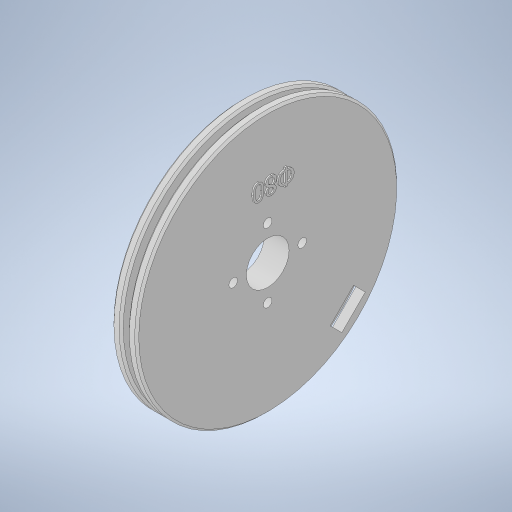
# Autodesk Inventor part: pully_shoulder_2_70
Saved by Autodesk Inventor 2024 (Build 280153000, 153)
## iProperties
Created: 2025-06-10
Part Number: pully_shoulder_2_70
Material: 一般
Document SubType Name: Modeling
Designer: HosodaLab2
Density: 1 g/cm^3
Appearance: 既定
Author: HosodaLab2
Autodesk Inventor part; units mm, degrees
ref_plane "YZ Plane" through (0, 0, 0) normal (1, 0, 0) x (0, 1, 0)
ref_plane "XZ Plane" through (0, 0, 0) normal (0, 1, 0) x (-1, 0, 0)
ref_plane "XY Plane" through (0, 0, 0) normal (0, 0, 1) x (1, 0, 0)
sketch "スケッチ1" plane through (0, 0, 0) normal (0, 1, 0) x (-1, 0, 0)
  circle A0 centre (0, 0) radius 40
  dimension "d0" = 80
  constraints: 1 centre point, 1 coincident
  measures "d0" diameter of A0
extrude "押し出し1" add sketch "スケッチ1" along normal blind 2.2
sketch "スケッチ2" plane through (0, 2.2, 0) normal (0, 1, 0) x (1, 0, 0)
  circle A0 centre (0, 0) radius 47.5
  line L0 (-3.6848, -24.5947) -> (4.9338, -24.5947) construction
  line L1 (4.9338, -24.5947) -> (4.9338, -28.142) construction
  line L2 (4.9338, -28.142) -> (-3.6848, -28.142) construction
  line L3 (-3.6848, -28.142) -> (-3.6848, -24.5947) construction
  dimension "d3" = 95
  constraints: 1 centre point, 1 coincident, 2 other
  measures "d3" diameter of A0
extrude "押し出し2" add sketch "スケッチ2" along normal blind 3.4
chamfer "面取り1" distance 0.75 angle 45 1 edges at (-47.5, 2.2, 0)
chamfer "面取り2" distance 0.75 angle 45 1 edges at (-47.5, 5.6, 0)
sketch "スケッチ3" plane through (0, 0, 0) normal (0, -1, 0) x (1, 0, 0)
  circle A0 centre (0, 0) radius 47.5
  dimension "d12" = 95
  constraints: 1 centre point, 1 coincident
  measures "d12" diameter of A0
extrude "押し出し3" add sketch "スケッチ3" along normal blind 3.4
chamfer "面取り3" distance 0.75 angle 45 1 edges at (-47.5, 0, 0)
chamfer "面取り4" distance 0.75 angle 45 1 edges at (-47.5, -3.4, 0)
sketch "スケッチ6" plane through (0, 5.6, 0) normal (0, 1, 0) x (1, 0, 0)
  circle A0 centre (0, 0) radius 7.65
  line L0 (0, 7.65) -> (46.8799, 7.65)
  circle A1 centre (0, 0) radius 47.5 projected
  line L1 (0, -7.65) -> (46.8799, -7.65)
  dimension "d39" = 15.3
  constraints: 4 end point, 4 point on circle, 1 centre point, 1 coincident, 1 horizontal, 1 parallel, 1 tangent
  measures "d39" diameter of A0
extrude "押し出し5" [suppressed]
chamfer "面取り7" [suppressed]
chamfer "面取り8" [suppressed]
chamfer "面取り9" [suppressed]
sketch "スケッチ7" plane through (0, 5.6, 0) normal (0, 1, 0) x (1, 0, 0)
  line L0 (-9.3358, -20.9354) -> (21.308, -20.9354) construction
  line L1 (21.308, -20.9354) -> (21.308, -27.5341) construction
  line L2 (21.308, -27.5341) -> (-9.3358, -27.5341) construction
  line L3 (-9.3358, -27.5341) -> (-9.3358, -20.9354) construction
  spline S0 degree 2 poles (-5.7914, -21.672) (-5.2131, -21.6818) (-4.2541, -22.0674) (-3.9377, -22.3887) knots 0 0 0 1 2 2 2
  spline S1 degree 2 poles (-3.9377, -22.3887) (-3.646, -22.6903) (-3.3247, -23.5356) (-3.3247, -24.0793) knots 0 0 0 1 2 2 2
  spline S2 degree 2 poles (-3.3247, -24.0793) (-3.3247, -24.6478) (-3.6708, -25.5228) (-3.9772, -25.8194) knots 0 0 0 1 2 2 2
  spline S3 degree 2 poles (-3.9772, -25.8194) (-4.3084, -26.1456) (-5.2773, -26.5065) (-5.7914, -26.5164) knots 0 0 0 1 2 2 2
  line L4 (-5.7914, -26.5164) -> (-5.7914, -27.2232)
  line L5 (-5.7914, -27.2232) -> (-6.6021, -27.2232)
  line L6 (-6.6021, -27.2232) -> (-6.6021, -26.5164)
  spline S4 degree 2 poles (-6.6021, -26.5164) (-7.1162, -26.5015) (-8.0802, -26.1654) (-8.4213, -25.8292) knots 0 0 0 1 2 2 2
  spline S5 degree 2 poles (-8.4213, -25.8292) (-8.7277, -25.5277) (-9.0688, -24.6429) (-9.0688, -24.0793) knots 0 0 0 1 2 2 2
  spline S6 degree 2 poles (-9.0688, -24.0793) (-9.0688, -23.5455) (-8.7426, -22.7002) (-8.446, -22.3937) knots 0 0 0 1 2 2 2
  spline S7 degree 2 poles (-8.446, -22.3937) (-8.1296, -22.0674) (-7.1805, -21.6868) (-6.6021, -21.672) knots 0 0 0 1 2 2 2
  line L7 (-6.6021, -21.672) -> (-6.6021, -21.0244)
  line L8 (-6.6021, -21.0244) -> (-5.7914, -21.0244)
  line L9 (-5.7914, -21.0244) -> (-5.7914, -21.672)
  spline S8 degree 2 poles (-5.7914, -25.9034) (-5.4207, -25.8935) (-4.8473, -25.6711) (-4.6594, -25.4832) knots 0 0 0 1 2 2 2
  spline S9 degree 2 poles (-4.6594, -25.4832) (-4.4073, -25.2361) (-4.17, -24.5292) (-4.17, -24.0447) knots 0 0 0 1 2 2 2
  spline S10 degree 2 poles (-4.17, -24.0447) (-4.17, -23.6394) (-4.3974, -22.972) (-4.6248, -22.7397) knots 0 0 0 1 2 2 2
  spline S11 degree 2 poles (-4.6248, -22.7397) (-4.8374, -22.5173) (-5.4009, -22.3047) (-5.7914, -22.2948) knots 0 0 0 1 2 2 2
  line L10 (-5.7914, -22.2948) -> (-5.7914, -25.9034)
  spline S12 degree 2 poles (-6.6021, -22.2948) (-6.9926, -22.2997) (-7.5562, -22.5222) (-7.7687, -22.7397) knots 0 0 0 1 2 2 2
  spline S13 degree 2 poles (-7.7687, -22.7397) (-7.9961, -22.9671) (-8.2235, -23.6493) (-8.2235, -24.0447) knots 0 0 0 1 2 2 2
  spline S14 degree 2 poles (-8.2235, -24.0447) (-8.2235, -24.5292) (-7.9862, -25.241) (-7.7341, -25.4832) knots 0 0 0 1 2 2 2
  spline S15 degree 2 poles (-7.7341, -25.4832) (-7.5463, -25.6612) (-6.9729, -25.8985) (-6.6021, -25.9034) knots 0 0 0 1 2 2 2
  line L11 (-6.6021, -25.9034) -> (-6.6021, -22.2948)
  spline S16 degree 2 poles (-0.7691, -27.3122) (-1.2238, -27.3122) (-1.9703, -27.0403) (-2.2323, -26.7882) knots 0 0 0 1 2 2 2
  spline S17 degree 2 poles (-2.2323, -26.7882) (-2.4893, -26.5411) (-2.7563, -25.8688) (-2.7563, -25.4882) knots 0 0 0 1 2 2 2
  spline S18 degree 2 poles (-2.7563, -25.4882) (-2.7563, -24.9938) (-2.2273, -24.1634) (-1.7231, -23.9162) knots 0 0 0 1 2 2 2
  line L12 (-1.7231, -23.9162) -> (-1.7231, -23.8915)
  spline S19 degree 2 poles (-1.7231, -23.8915) (-2.173, -23.6295) (-2.608, -23.0066) (-2.608, -22.542) knots 0 0 0 1 2 2 2
  spline S20 degree 2 poles (-2.608, -22.542) (-2.608, -21.8549) (-1.5699, -20.9354) (-0.7691, -20.9354) knots 0 0 0 1 2 2 2
  spline S21 degree 2 poles (-0.7691, -20.9354) (0.0614, -20.9354) (1.0649, -21.8054) (1.0649, -22.4876) knots 0 0 0 1 2 2 2
  spline S22 degree 2 poles (1.0649, -22.4876) (1.0649, -22.8979) (0.5854, -23.6987) (0.1356, -23.9261) knots 0 0 0 1 2 2 2
  line L13 (0.1356, -23.9261) -> (0.1356, -23.9508)
  spline S23 degree 2 poles (0.1356, -23.9508) (0.6694, -24.198) (1.2181, -24.9098) (1.2181, -25.4733) knots 0 0 0 1 2 2 2
  spline S24 degree 2 poles (1.2181, -25.4733) (1.2181, -26.2544) (0.0812, -27.3122) (-0.7691, -27.3122) knots 0 0 0 1 2 2 2
  spline S25 degree 2 poles (0.3778, -25.5524) (0.3778, -25.1767) (0.0812, -24.7318) (-0.339, -24.5044) knots 0 0 0 1 2 2 2
  spline S26 degree 2 poles (-0.339, -24.5044) (-0.4774, -24.4254) (-0.9421, -24.2425) (-1.2337, -24.1238) knots 0 0 0 1 2 2 2
  spline S27 degree 2 poles (-1.2337, -24.1238) (-1.5699, -24.3463) (-1.9307, -25.0087) (-1.9307, -25.4288) knots 0 0 0 1 2 2 2
  spline S28 degree 2 poles (-1.9307, -25.4288) (-1.9307, -25.9825) (-1.2634, -26.7042) (-0.7592, -26.7042) knots 0 0 0 1 2 2 2
  spline S29 degree 2 poles (-0.7592, -26.7042) (-0.2451, -26.7042) (0.3778, -26.0863) (0.3778, -25.5524) knots 0 0 0 1 2 2 2
  spline S30 degree 2 poles (0.2641, -22.4975) (0.2641, -22.0872) (-0.2846, -21.5385) (-0.774, -21.5385) knots 0 0 0 1 2 2 2
  spline S31 degree 2 poles (-0.774, -21.5385) (-1.2189, -21.5385) (-1.7874, -22.0279) (-1.7874, -22.448) knots 0 0 0 1 2 2 2
  spline S32 degree 2 poles (-1.7874, -22.448) (-1.7874, -22.7496) (-1.4957, -23.1698) (-1.2041, -23.3378) knots 0 0 0 1 2 2 2
  spline S33 degree 2 poles (-1.2041, -23.3378) (-1.0805, -23.407) (-0.5565, -23.6493) (-0.3439, -23.7185) knots 0 0 0 1 2 2 2
  spline S34 degree 2 poles (-0.3439, -23.7185) (0.012, -23.4466) (0.2641, -22.8682) (0.2641, -22.4975) knots 0 0 0 1 2 2 2
  spline S35 degree 2 poles (5.761, -24.1238) (5.761, -25.765) (4.8069, -27.3023) (3.8134, -27.3023) knots 0 0 0 1 2 2 2
  spline S36 degree 2 poles (3.8134, -27.3023) (2.8049, -27.3023) (1.8608, -25.7353) (1.8608, -24.1288) knots 0 0 0 1 2 2 2
  spline S37 degree 2 poles (1.8608, -24.1288) (1.8608, -22.4777) (2.8148, -20.9502) (3.8134, -20.9502) knots 0 0 0 1 2 2 2
  spline S38 degree 2 poles (3.8134, -20.9502) (4.8168, -20.9502) (5.761, -22.5321) (5.761, -24.1238) knots 0 0 0 1 2 2 2
  spline S39 degree 2 poles (4.713, -25.9825) (4.8317, -25.6809) (4.9305, -24.7516) (4.9305, -24.1238) knots 0 0 0 1 2 2 2
  spline S40 degree 2 poles (4.9305, -24.1238) (4.9305, -23.496) (4.8317, -22.5716) (4.7081, -22.2602) knots 0 0 0 1 2 2 2
  spline S41 degree 2 poles (4.7081, -22.2602) (4.5845, -21.9488) (4.1544, -21.6275) (3.8134, -21.6275) knots 0 0 0 1 2 2 2
  spline S42 degree 2 poles (3.8134, -21.6275) (3.4723, -21.6275) (3.0323, -21.9488) (2.9038, -22.2701) knots 0 0 0 1 2 2 2
  spline S43 degree 2 poles (2.9038, -22.2701) (2.7802, -22.5815) (2.6912, -23.5306) (2.6912, -24.1288) knots 0 0 0 1 2 2 2
  spline S44 degree 2 poles (2.6912, -24.1288) (2.6912, -24.7714) (2.7703, -25.6315) (2.8988, -25.9677) knots 0 0 0 1 2 2 2
  spline S45 degree 2 poles (2.8988, -25.9677) (3.0175, -26.284) (3.4574, -26.6251) (3.8134, -26.6251) knots 0 0 0 1 2 2 2
  spline S46 degree 2 poles (3.8134, -26.6251) (4.1495, -26.6251) (4.5894, -26.3038) (4.713, -25.9825) knots 0 0 0 1 2 2 2
  point P0 (0, 0)
  constraints: 2 other
extrude "押し出し6" add sketch "スケッチ7" along normal blind 0.5
sketch "スケッチ8" plane through (0, 5.6, 0) normal (0, 1, 0) x (1, 0, 0)
  circle A0 centre (0, 0) radius 46.75 projected
  line L0 (0, 0) -> (-33.5876, 33.5876) construction
  circle A1 centre (0, 0) radius 47.5 projected
  line L1 (0, 0) -> (47.5, 0) construction
  line L2 (-26.8701, 35.3553) -> (-35.3553, 26.8701)
  line L3 (-35.3553, 26.8701) -> (-31.1127, 22.6274)
  line L4 (-31.1127, 22.6274) -> (-22.6274, 31.1127)
  line L5 (-22.6274, 31.1127) -> (-26.8701, 35.3553)
  line L6 (-26.8701, 35.3553) -> (-31.1127, 22.6274) construction
  line L7 (-35.3553, 26.8701) -> (-22.6274, 31.1127) construction
  point P0 (-28.9914, 28.9914)
  dimension "d83" = 135
  dimension "d84" = 6
  dimension "d85" = 12
  dimension "d86" = 38
  constraints: 16 end point, 2 midpoint, 2 parallel, 2 perpendicular, 1 equal length, 1 horizontal, 1 point on line, 2 other
  measures "d83" angle of L1 L0
  measures "d84" distance of L3.end L2.end
  measures "d85" distance between parallel lines of L5 L3
  measures "d86" distance from line of L4 point (0, 0)
extrude "押し出し7" cut sketch "スケッチ8" against normal blind 10 contours L5 L4 L3 L2
sketch "スケッチ9" plane through (0, 5.6, 0) normal (0, 1, 0) x (1, 0, 0)
  point P0 (0, 0)
  point P1 (0, 0)
  constraints: 1 coincident
hole "穴2" at (0, 5.6, 0) direction (0, -1, 0) diameter 15.5 end through all
sketch "スケッチ10" plane through (0, 5.6, 0) normal (0, 1, 0) x (1, 0, 0)
  circle A0 centre (0, 0) radius 12.5 construction
  point P0 (0, -12.5)
  point P1 (12.5, 0)
  point P2 (0, 12.5)
  point P3 (-12.5, 0)
  dimension "d67" = 25
  dimension "d81" = 360
  constraints: 1 coincident, 1 vertical alignment, 7 other
hole "穴3" at (0, 5.6, 12.5) at (-12.5, 5.6, 0) at (0, 5.6, -12.5) at (12.5, 5.6, 0) direction (0, -1, 0) diameter 3.2 end through all
